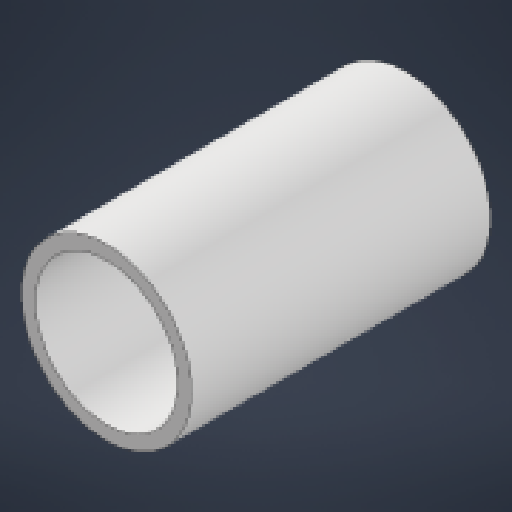
# Autodesk Inventor part: ServoSpacer
Saved by Autodesk Inventor 2024.1 (Build 281209000, 209)
## iProperties
Created: 2023-11-16
Part Number: ServoSpacer
Material: Generic
Document SubType Name: Modeling
Designer: Brandon
Density: 1 g/cm^3
Appearance: Default
Author: Brandon
Autodesk Inventor part; units mm, degrees
ref_plane "YZ Plane" through (0, 0, 0) normal (1, 0, 0) x (0, 1, 0)
ref_plane "XZ Plane" through (0, 0, 0) normal (0, 1, 0) x (-1, 0, 0)
ref_plane "XY Plane" through (0, 0, 0) normal (0, 0, 1) x (1, 0, 0)
sketch "Sketch1" plane through (0, 0, 0) normal (0, 0, 1) x (1, 0, 0)
  arc A0 (13.554, -7.5586) -> (10.818, -7.5586) centre (12.186, -6.0655) ccw projected
  arc A1 (12.5997, -7.5323) -> (11.7723, -7.5323) centre (12.186, -6.0655) ccw projected
  arc A2 (13.5197, -7.5211) -> (10.8523, -7.5211) centre (12.186, -6.0655) ccw
  arc A3 (12.6342, -7.6545) -> (11.7378, -7.6545) centre (12.186, -6.0655) ccw
  circle A4 centre (12.186, -6.0655) radius 1.651
  circle A5 centre (12.186, -6.0655) radius 1.9742
  point P0 (0, 0)
  dimension "d0" = 0.0508
  dimension "d1" = 0.127
  constraints: 4 point on circle, 2 centre point, 2 coincident, 6 other
  measures "d0" radial gap between concentric circles of A0 A2
  measures "d1" radial gap between concentric circles of A1 A3
extrude "Extrusion1" add sketch "Sketch1" along normal blind 6.9342
body "Solid1"
